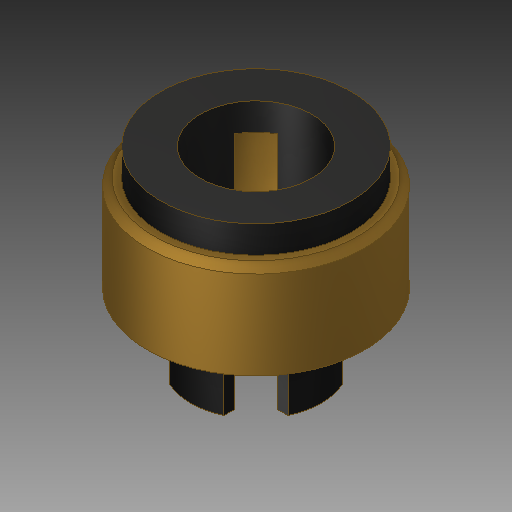
# Autodesk Inventor part: Collet
Saved by Autodesk Inventor 2019 (Build 230136000, 136)
## iProperties
Created: 2018-09-16
Part Number: Collet
Material: Acetal Resin, Black
Document SubType Name: Modeling
Designer: Ax
Density: 1.425 g/cm^3
Appearance: Brass - Satin
Mass: 0.220215 g
Surface Area: 3.06694 cm^2
Volume: 0.154537 cm^3
Author: Ax
Autodesk Inventor part; units mm, degrees
ref_plane "YZ Plane" through (0, 0, 0) normal (1, 0, 0) x (0, 1, 0)
ref_plane "XZ Plane" through (0, 0, 0) normal (0, 1, 0) x (-1, 0, 0)
ref_plane "XY Plane" through (0, 0, 0) normal (0, 0, 1) x (1, 0, 0)
sketch "Sketch1" plane through (0, 0, 0) normal (0, 1, 0) x (-1, 0, 0)
  circle A0 centre (0, 0) radius 2.4
  circle A1 centre (0, 0) radius 4
  dimension "d0" = 8
  dimension "d1" = 4.8
  constraints: 2 centre point, 2 coincident
  measures "d0" diameter of A1
  measures "d1" diameter of A0
extrude "Extrusion1" add sketch "Sketch1" along normal blind 3.5
chamfer "Chamfer1" distance 0.25 angle 45 1 edges at (4, 3.5, 0)
sketch "Sketch2" plane through (0, 3.5, 0) normal (0, 1, 0) x (1, 0, 0)
  circle A0 centre (0, 0) radius 2.05
  circle A1 centre (0, 0) radius 3.5
  dimension "d7" = 4.1
  dimension "d8" = 7
  constraints: 2 centre point, 2 coincident
  measures "d7" diameter of A0
  measures "d8" diameter of A1
extrude "Extrusion2" add sketch "Sketch2" along normal blind 1
sketch "Sketch3" plane through (0, 3.5, 0) normal (0, -1, 0) x (1, 0, 0)
  arc A0 (-1.0733, -2.1466) -> (1, -2.1817) centre (0, 0) ccw
  arc A1 (-1, -1.7896) -> (1, -1.7896) centre (0, 0) ccw
  line L0 (-1, -1.7896) -> (-1, -2.1817)
  line L1 (1, -1.7896) -> (1, -2.1817)
  line L2 (0, 0) -> (0, -5.6159) construction
  dimension "d11" = 2.05
  dimension "d13" = 2.4
  dimension "d14" = 2
  constraints: 6 end point, 6 point on circle, 2 centre point, 2 coincident, 2 vertical, 1 parallel, 1 other
  measures "d11" radius of A1
  measures "d13" radius of A0
  measures "d14" distance of L1.start L0.start
extrude "Extrusion3" add sketch "Sketch3" along normal blind 6
pattern_circular "Circular Pattern1" count 4 over 360 about axis through (0, -10, 0) along (0, 1, 0) of "Extrusion3"
body "Solid1"
